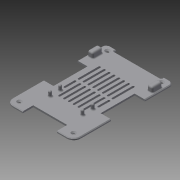
# Autodesk Inventor part: Deckel2_Motor2_liegend
Saved by Autodesk Inventor 2015 (Build 190159000, 159)
## iProperties
Created: 2015-03-02
Part Number: Deckel2_Motor2_liegend
Material: Generisch
Document SubType Name: Modeling
Designer: TowerSebi
Density: 1 g/cm^3
Appearance: Vorgabe
Author: TowerSebi
Autodesk Inventor part; units mm, degrees
ref_plane "YZ Plane" through (0, 0, 0) normal (1, 0, 0) x (0, 1, 0)
ref_plane "XZ Plane" through (0, 0, 0) normal (0, 1, 0) x (-1, 0, 0)
ref_plane "XY Plane" through (0, 0, 0) normal (0, 0, 1) x (1, 0, 0)
sketch "Skizze1" plane through (0, 0, 0) normal (0, 0, 1) x (1, 0, 0)
  line L0 (0, 0) -> (100, 0)
  line L1 (100, 0) -> (100, 145)
  line L2 (0, 145) -> (0, 0)
  arc A0 (100, 145) -> (0, 145) centre (50, 69.1667) ccw
  dimension "d0" = 145
  dimension "d1" = 100
  constraints: 6 end point, 2 point on circle, 1 centre point, 1 horizontal, 1 parallel, 1 perpendicular
  measures "d0" distance of L2.start L0.start
  measures "d1" distance of L1.end L2.start
extrude "Extrusion1" add sketch "Skizze1" along normal blind 2.5
fillet "Rundung2" radius 10 2 edges at (100, 0, 1.25) (0, 0, 1.25)
fillet "Rundung3" radius 5 2 edges at (100, 145, 1.25) (0, 145, 1.25)
sketch "Skizze3" plane through (0, 0, 0) normal (0, 0, -1) x (-1, 0, 0)
  line L0 (-10, 0) -> (-90, 0) projected
  line L1 (0, 142.2581) -> (0, 10) projected
  circle A0 centre (-90, 10) radius 1.5
  circle A1 centre (-10, 10) radius 1.5
  circle A2 centre (-10, 140) radius 1.5
  circle A3 centre (-90, 140) radius 1.5
  point P0 (0, 0)
  dimension "d12" = 3
  dimension "d14" = 3
  dimension "d19" = 3
  dimension "d22" = 3
  dimension "d23" = 140
  dimension "d25" = 140
  dimension "d30" = 10
  dimension "d33" = 10
  dimension "d34" = 90
  dimension "d37" = 10
  dimension "d42" = 90
  dimension "d44" = 10
  constraints: 4 centre point
  measures "d12" diameter of A3
  measures "d14" diameter of A2
  measures "d19" diameter of A0
  measures "d22" diameter of A1
  measures "d23" distance from line of L0 A3.centre
  measures "d25" distance from line of L0 A2.centre
  measures "d30" distance from line of L0 A0.centre
  measures "d33" distance from line of L0 A1.centre
  measures "d34" distance from line of L1 A0.centre
  measures "d37" distance of L1.end A1.centre
  measures "d42" distance from line of A3.centre L1
  measures "d44" distance from line of L1 A2.centre
extrude "Extrusion2" cut sketch "Skizze3" against normal up to next
sketch "Skizze10" plane through (0, 0, 2.5) normal (0, 0, 1) x (1, 0, 0)
  line L0 (0, 142.2581) -> (0, 10) projected
  line L1 (10, 0) -> (90, 0) projected
  line L2 (100, 10) -> (100, 142.2581) projected
  arc A0 (97.6214, 146.5159) -> (2.3786, 146.5159) centre (50, 69.1667) ccw projected
  line L3 (5, 110) -> (20, 110)
  line L4 (14.8779, 148) -> (14.8779, 144)
  line L5 (14.8779, 144) -> (85.1221, 144)
  line L6 (85.1221, 144) -> (85.1221, 148)
  line L7 (14.8779, 148) -> (4.8779, 148)
  line L8 (85.1221, 148) -> (95.1221, 148)
  line L9 (0, 105.05) -> (15.1, 105.05)
  line L10 (15.1, 105.05) -> (15.1, 54.95)
  line L11 (15.1, 54.95) -> (0, 54.95)
  line L12 (100, 105.05) -> (84.9, 105.05)
  line L13 (84.9, 105.05) -> (84.9, 54.95)
  line L14 (84.9, 54.95) -> (100, 54.95)
  line L15 (24.95, 0) -> (24.95, 15.1)
  line L16 (24.95, 15.1) -> (75.05, 15.1)
  line L17 (75.05, 15.1) -> (75.05, 0)
  point P0 (0, 0)
  dimension "d154" = 4
  dimension "d155" = 4
  dimension "d162" = 15.1
  dimension "d163" = 50.1
  dimension "d164" = 15.1
  dimension "d165" = 50.1
  dimension "d167" = 4.95
  dimension "d168" = 15.1
  dimension "d171" = 50.1
  dimension "d191" = 10
  dimension "d192" = 10
  constraints: 30 end point, 6 perpendicular, 6 point on line, 2 parallel, 2 point on circle
  measures "d154" distance between parallel lines of L5 L7
  measures "d155" distance between parallel lines of L5 L8
  measures "d162" distance of L9.start L9.end
  measures "d163" distance of L9.end L10.end
  measures "d164" distance of L12.start L12.end
  measures "d165" distance of L12.end L13.end
  measures "d167" distance between parallel lines of L3 L9
  measures "d168" distance of L15.start L15.end
  measures "d171" distance of L15.end L16.end
  measures "d191" distance of L4.start L7.end
  measures "d192" distance of L6.end L8.end
extrude "Extrusion11" cut sketch "Skizze10" against normal up to next
fillet "Rundung9" radius 1 4 edges at (14.8779, 148, 1.25) (85.1221, 148, 1.25) (85.1221, 144, 1.25) (14.8779, 144, 1.25)
sketch "Skizze12" plane through (0, 0, 2.5) normal (0, 0, 1) x (1, 0, 0)
  line L0 (85.1221, 147) -> (85.1221, 145) projected
  line L1 (0, 142.2581) -> (0, 105.05) projected
  line L2 (10, 0) -> (24.95, 0) projected
  line L3 (25, 113) -> (25, 83) construction
  line L4 (23.5, 113) -> (23.5, 83)
  line L5 (26.5, 83) -> (26.5, 113)
  arc A0 (26.5, 113) -> (23.5, 113) centre (25, 113) ccw
  arc A1 (23.5, 83) -> (26.5, 83) centre (25, 83) ccw
  line L6 (25, 77) -> (25, 47) construction
  line L7 (23.5, 77) -> (23.5, 47)
  line L8 (26.5, 47) -> (26.5, 77)
  arc A2 (26.5, 77) -> (23.5, 77) centre (25, 77) ccw
  arc A3 (23.5, 47) -> (26.5, 47) centre (25, 47) ccw
  point P0 (0, 0)
  point P1 (25, 98)
  point P2 (25, 62)
  dimension "d239" = 30
  dimension "d240" = 30
  dimension "d241" = 6
  dimension "d242" = 3
  dimension "d243" = 3
  dimension "d244" = 47
  dimension "d245" = 25
  dimension "d246" = 25
  constraints: 16 end point, 8 point on circle, 8 tangent, 4 centre point, 4 parallel, 2 midpoint
  measures "d239" distance of L3.start L3.end
  measures "d240" distance of L6.end L6.start
  measures "d241" distance of L6.start L3.end
  measures "d242" distance between parallel lines of L4 L5
  measures "d243" distance between parallel lines of L7 L8
  measures "d244" distance from line of L2 L6.end
  measures "d245" distance from line of L1 L3.start
  measures "d246" distance from line of L1 L6.start
extrude "Extrusion13" cut sketch "Skizze12" against normal up to next
pattern_linear "Rechteckige Anordnung1" count 8 spacing 7.15 along (1, 0, 0) of "Extrusion13"
chamfer "Fase1" [suppressed]
sketch "Skizze13" plane through (0, 0, 2.5) normal (0, 0, 1) x (1, 0, 0)
  line L0 (24, 41) -> (28, 41)
  line L1 (28, 41) -> (28, 37)
  line L2 (28, 37) -> (24, 37)
  line L3 (24, 37) -> (24, 41)
  line L4 (72, 41) -> (76, 41)
  line L5 (76, 41) -> (76, 37)
  line L6 (76, 37) -> (72, 37)
  line L7 (72, 37) -> (72, 41)
  line L8 (24, 56) -> (28, 56)
  line L9 (28, 56) -> (28, 52)
  line L10 (28, 52) -> (24, 52)
  line L11 (24, 52) -> (24, 56)
  line L12 (72, 52) -> (76, 52)
  line L13 (76, 52) -> (76, 56)
  line L14 (76, 56) -> (72, 56)
  line L15 (72, 56) -> (72, 52)
  line L16 (10, 0) -> (24.95, 0) projected
  line L17 (75.05, 0) -> (90, 0) projected
  line L18 (0, 54.95) -> (0, 10) projected
  line L19 (100, 10) -> (100, 54.95) projected
  point P0 (0, 0)
  dimension "d291" = 4
  dimension "d292" = 4
  dimension "d293" = 4
  dimension "d294" = 4
  dimension "d297" = 4
  dimension "d298" = 4
  dimension "d299" = 41
  dimension "d300" = 41
  dimension "d301" = 24
  dimension "d302" = 24
  dimension "d303" = 4
  dimension "d304" = 4
  dimension "d305" = 24
  dimension "d306" = 24
  dimension "d307" = 11
  dimension "d308" = 11
  constraints: 32 end point, 8 parallel, 4 horizontal, 4 perpendicular
  measures "d291" distance of L1.end L2.end
  measures "d292" distance of L5.end L6.end
  measures "d293" distance of L12.start L12.end
  measures "d294" distance of L9.end L10.end
  measures "d297" distance of L2.end L0.start
  measures "d298" distance of L4.end L5.end
  measures "d299" distance between parallel lines of L17 L4
  measures "d300" distance between parallel lines of L16 L0
  measures "d301" distance between parallel lines of L18 L3
  measures "d302" distance between parallel lines of L19 L5
  measures "d303" distance of L8.end L9.end
  measures "d304" distance of L12.end L13.end
  measures "d305" distance between parallel lines of L19 L13
  measures "d306" distance between parallel lines of L18 L11
  measures "d307" distance between parallel lines of L12 L4
  measures "d308" distance between parallel lines of L0 L10
extrude "Extrusion14" add sketch "Skizze13" along normal blind 8
fillet "Rundung10" radius 2 8 edges at (26, 37, 10.5) (26, 41, 10.5) (26, 52, 10.5) (26, 56, 10.5) (74, 37, 10.5) (74, 41, 10.5) (74, 52, 10.5) (74, 56, 10.5)
sketch "Skizze14" plane through (0, 0, 2.5) normal (0, 0, 1) x (1, 0, 0)
  line L0 (28, 52) -> (26.5, 52) projected
  line L1 (26.5, 77) -> (26.5, 47) projected
  arc A0 (23.5, 47) -> (26.5, 47) centre (25, 47) ccw projected
  line L2 (23.5, 47) -> (23.5, 77) projected
  arc A1 (26.5, 77) -> (23.5, 77) centre (25, 77) ccw projected
  line L3 (26.5, 77) -> (26.5, 47) projected
  line L4 (26.5, 56) -> (28, 56) projected
  line L5 (28, 56) -> (28, 52) projected
  line L6 (72, 56) -> (73.55, 56) projected
  line L7 (73.55, 47) -> (73.55, 77) projected
  arc A2 (76.55, 77) -> (73.55, 77) centre (75.05, 77) ccw projected
  line L8 (76.55, 77) -> (76.55, 47) projected
  arc A3 (73.55, 47) -> (76.55, 47) centre (75.05, 47) ccw projected
  line L9 (73.55, 47) -> (73.55, 77) projected
  line L10 (73.55, 52) -> (72, 52) projected
  line L11 (72, 52) -> (72, 56) projected
  line L12 (25, 77) -> (25, 62) construction
  line L13 (23.5, 77) -> (23.5, 62)
  line L14 (26.5, 62) -> (26.5, 77)
  arc A4 (26.5, 77) -> (23.5, 77) centre (25, 77) ccw
  arc A5 (23.5, 62) -> (26.5, 62) centre (25, 62) ccw
  line L15 (75.05, 77) -> (75.05, 62) construction
  line L16 (73.55, 77) -> (73.55, 62)
  line L17 (76.55, 62) -> (76.55, 77)
  arc A6 (76.55, 77) -> (73.55, 77) centre (75.05, 77) ccw
  arc A7 (73.55, 62) -> (76.55, 62) centre (75.05, 62) ccw
  circle A8 centre (25, 47) radius 1.5
  circle A9 centre (75.05, 47) radius 1.5
  line L18 (26.5, 62) -> (26.5, 47)
  line L19 (23.5, 47) -> (23.5, 62)
  line L20 (76.55, 62) -> (76.55, 47)
  line L21 (73.55, 47) -> (73.55, 62)
  point P0 (0, 0)
  point P1 (25, 69.5)
  point P2 (75.05, 69.5)
  dimension "d312" = 15
  dimension "d313" = 15
  constraints: 24 end point, 8 point on circle, 8 tangent, 6 centre point, 6 parallel, 2 coincident, 2 concentric, 2 midpoint
  measures "d312" distance of L12.start L12.end
  measures "d313" distance of L15.end L15.start
extrude "Extrusion15" add sketch "Skizze14" against normal blind 2.5 contours L0 L1 L4 L5 | L1 A8 L2 A5 | A0 A8 | L6 L7 L10 L11 | L7 A7 L8 A9 | A9 A3
fillet "Rundung11" radius 2 24 edges at (76, 56, 5.5) (76, 52, 5.5) (76, 52.5858, 9.9142) (72, 52, 5.5) (72, 56, 5.5) (72, 52.5858, 9.9142) (76, 41, 5.5) (76, 37, 5.5) (76, 37.5858, 9.9142) (72, 37, 5.5) (72, 41, 5.5) (72, 37.5858, 9.9142) (28, 56, 5.5) (28, 52, 5.5) (28, 52.5858, 9.9142) (28, 41, 5.5) (28, 37, 5.5) (28, 37.5858, 9.9142) (24, 52, 5.5) (24, 56, 5.5) (24, 52.5858, 9.9142) (24, 37, 5.5) (24, 41, 5.5) (24, 37.5858, 9.9142)
fillet "Rundung12" radius 2 12 edges at (74, 56, 2.5) (75.4142, 55.4142, 2.5) (76, 54, 2.5) (74, 41, 2.5) (75.4142, 40.4142, 2.5) (76, 39, 2.5) (26, 41, 2.5) (27.4142, 40.4142, 2.5) (28, 39, 2.5) (28, 54, 2.5) (27.4142, 55.4142, 2.5) (26, 56, 2.5)
sketch "Skizze15" plane through (0, 0, 2.5) normal (0, 0, 1) x (1, 0, 0)
  line L0 (0, 142.2581) -> (0, 105.05) projected
  line L1 (0, 105.05) -> (15.1, 105.05) projected
  line L2 (15.1, 105.05) -> (15.1, 54.95) projected
  line L3 (15.1, 54.95) -> (0, 54.95) projected
  line L4 (0, 54.95) -> (0, 10) projected
  line L5 (10, 0) -> (24.95, 0) projected
  line L6 (24.95, 0) -> (24.95, 15.1) projected
  line L7 (24.95, 15.1) -> (75.05, 15.1) projected
  line L8 (75.05, 15.1) -> (75.05, 0) projected
  line L9 (75.05, 0) -> (90, 0) projected
  line L10 (100, 10) -> (100, 54.95) projected
  line L11 (100, 54.95) -> (84.9, 54.95) projected
  line L12 (84.9, 54.95) -> (84.9, 105.05) projected
  line L13 (84.9, 105.05) -> (100, 105.05) projected
  line L14 (100, 105.05) -> (100, 142.2581) projected
  line L15 (95.1221, 148) -> (86.1221, 148) projected
  line L16 (0, 105.1) -> (15.2, 105.1)
  line L17 (15.2, 105.1) -> (15.2, 54.9)
  line L18 (15.2, 54.9) -> (0, 54.9)
  line L19 (100, 105.1) -> (84.8, 105.1)
  line L20 (84.8, 105.1) -> (84.8, 54.9)
  line L21 (84.8, 54.9) -> (100, 54.9)
  line L22 (24.9, 0) -> (24.9, 15.2)
  line L23 (24.9, 15.2) -> (75.1, 15.2)
  line L24 (75.1, 15.2) -> (75.1, 0)
  point P0 (0, 0)
  point P1 (0.5, 105.05)
  point P2 (0.5, 54.95)
  point P3 (24.95, 0.5)
  point P4 (75.05, 0.5)
  point P5 (99.5, 54.95)
  point P6 (99.5, 105.05)
  dimension "d318" = 0.05
  dimension "d319" = 0.05
  dimension "d320" = 0.1
  dimension "d321" = 0.05
  dimension "d322" = 0.05
  dimension "d323" = 0.1
  dimension "d324" = 0.05
  dimension "d325" = 0.05
  dimension "d326" = 0.1
  constraints: 18 end point, 6 point on line, 5 perpendicular, 4 parallel
  measures "d318" distance between parallel lines of L1 L16
  measures "d319" distance between parallel lines of L3 L18
  measures "d320" distance between parallel lines of L17 L2
  measures "d321" distance between parallel lines of L6 L22
  measures "d322" distance between parallel lines of L8 L24
  measures "d323" distance between parallel lines of L23 L7
  measures "d324" distance between parallel lines of L11 L21
  measures "d325" distance between parallel lines of L13 L19
  measures "d326" distance between parallel lines of L12 L20
extrude "Extrusion16" cut sketch "Skizze15" against normal up to next
chamfer "Fase2" distance 1 angle 45 21 edges at (0, 32.45, 2.5) (2.9289, 2.9289, 2.5) (17.45, 0, 2.5) (97.0711, 2.9289, 2.5) (82.55, 0, 2.5) (100, 32.45, 2.5) (100, 123.6791, 2.5) (99.365, 144.6967, 2.5) (96.3776, 147.2679, 2.5) (0, 123.6791, 2.5) (0.635, 144.6967, 2.5) (3.6224, 147.2679, 2.5) (50, 144, 2.5) (15.1708, 144.2929, 2.5) (14.8779, 146, 2.5) (14.5851, 147.7071, 2.5) (9.3779, 148, 2.5) (84.8292, 144.2929, 2.5) (85.1221, 146, 2.5) (85.4149, 147.7071, 2.5) (90.6221, 148, 2.5)
hole "Bohrung6" at (10, 10, 2.5) direction (0, 0, -1) diameter 3.4 end through all countersink diameter 7 countersink angle 90 clearance for "Senkschraube mit Linsenkopf ISO 2010" size "M3" standard "DIN"
hole "Bohrung7" at (90, 10, 2.5) direction (0, 0, -1) diameter 3.4 end through all countersink diameter 7 countersink angle 90 clearance for "Senkschraube mit Linsenkopf ISO 2010" size "M3" standard "DIN"
hole "Bohrung8" at (90, 140, 2.5) direction (0, 0, -1) diameter 3.4 end through all countersink diameter 7 countersink angle 90 clearance for "Senkschraube mit Linsenkopf ISO 2010" size "M3" standard "DIN"
hole "Bohrung9" at (10, 140, 2.5) direction (0, 0, -1) diameter 3.4 end through all countersink diameter 7 countersink angle 90 clearance for "Senkschraube mit Linsenkopf ISO 2010" size "M3" standard "DIN"
sketch "Skizze17" plane through (0, 0, 2.5) normal (0, 0, 1) x (1, 0, 0)
  line L0 (2, 133) -> (10, 133)
  line L1 (10, 133) -> (10, 118)
  line L2 (10, 118) -> (2, 118)
  line L3 (2, 118) -> (2, 133)
  line L4 (90, 133) -> (98, 133)
  line L5 (98, 133) -> (98, 118)
  line L6 (98, 118) -> (90, 118)
  line L7 (90, 118) -> (90, 133)
  line L8 (13.8779, 148) -> (4.8779, 148) projected
  line L9 (95.1221, 148) -> (86.1221, 148) projected
  line L10 (0, 142.2581) -> (0, 105.1) projected
  line L11 (100, 105.1) -> (100, 142.2581) projected
  point P0 (0, 0)
  dimension "d378" = 8
  dimension "d379" = 8
  dimension "d380" = 15
  dimension "d381" = 15
  dimension "d382" = 15
  dimension "d383" = 15
  dimension "d384" = 2
  dimension "d385" = 2
  constraints: 16 end point, 4 parallel, 2 horizontal, 2 perpendicular
  measures "d378" distance of L0.start L0.end
  measures "d379" distance of L4.start L4.end
  measures "d380" distance of L2.end L0.start
  measures "d381" distance of L6.end L4.start
  measures "d382" distance between parallel lines of L8 L0
  measures "d383" distance between parallel lines of L9 L4
  measures "d384" distance between parallel lines of L10 L3
  measures "d385" distance between parallel lines of L11 L5
extrude "Extrusion18" add sketch "Skizze17" along normal blind 8
fillet "Rundung16" radius 2.5 4 edges at (10, 125.5, 10.5) (2, 125.5, 10.5) (98, 125.5, 10.5) (90, 125.5, 10.5)
fillet "Rundung17" radius 2.5 12 edges at (97.2678, 118, 9.7678) (98, 118, 5.25) (90, 118, 5.25) (90, 133, 5.25) (98, 133, 5.25) (97.2678, 133, 9.7678) (2, 133, 5.25) (10, 133, 5.25) (9.2678, 133, 9.7678) (10, 118, 5.25) (2, 118, 5.25) (9.2678, 118, 9.7678)
fillet "Rundung18" radius 1.5 8 edges at (9.2678, 118.7322, 2.5) (2, 125.5, 2.5) (2.7322, 132.2678, 2.5) (10, 125.5, 2.5) (97.2678, 118.7322, 2.5) (90, 125.5, 2.5) (90.7322, 132.2678, 2.5) (98, 125.5, 2.5)
